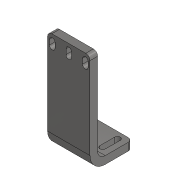
# Autodesk Inventor part: TL20240701-10200AT-005
Saved by Autodesk Inventor 2022.5 (Build 265521000, 521)
## iProperties
Category: ANTI BACK ASSY
Company: 현대트랜시스(대유)
RuleStatus: InUse
Part Number: TL20240701-10200AT-005
Project: SW-PJT
Checked By: 김형민
Engr Approved By: 김시현
User Status: 1
Material: SS400
Description: 0
Document SubType Name: Modeling
Mfg Approved By: 호상태
Designer: USER106
Stock Number: 005
Density: 7.85 g/cm^3
Appearance: Plating Zinc White
Detail Description: Processed products
Title: BRACKET
Subject: SW차종 시트조립라인
Author: USER106
Revision Number: A
Autodesk Inventor part; units mm, degrees
ref_plane "YZ Plane" through (0, 0, 0) normal (1, 0, 0) x (0, 1, 0)
ref_plane "XZ Plane" through (0, 0, 0) normal (0, 1, 0) x (-1, 0, 0)
ref_plane "XY Plane" through (0, 0, 0) normal (0, 0, 1) x (1, 0, 0)
sketch "Sketch2" plane through (0, 0, 0) normal (1, 0, 0) x (0, 1, 0)
  line L0 (-25, 60) -> (-25, -60)
  line L1 (-25, -60) -> (25, -60)
  line L2 (-16, 60) -> (-16, -51)
  line L3 (-16, -51) -> (25, -51)
  line L4 (-16, 60) -> (-25, 60)
  line L5 (25, -60) -> (25, -51)
  point P0 (0, 0)
  point P1 (-25, 0)
  point P2 (0, -60)
  dimension "d1" = 120
  dimension "d2" = 50
  dimension "t" = 9
  constraints: 12 end point, 2 midpoint, 2 perpendicular, 2 vertical, 1 horizontal, 1 horizontal alignment, 1 vertical alignment, 1 other
  measures "d1" distance of L0.start L0.end
  measures "d2" distance of L0.end L1.end
  measures "t" distance between parallel lines of L0 L2
extrude "Extrusion1" add sketch "Sketch2" along normal mid plane 50
fillet "Fillet1" radius 9 1 edges at (0, -16, -51)
fillet "Fillet1" radius 18 1 edges at (0, -25, -60)
sketch "Sketch3" plane through (-25, -25, 60) normal (0, -1, 0) x (1, 0, 0)
  line L0 (50, 0) -> (0, 0) projected
  line L1 (0, -102) -> (0, 0) projected
  line L2 (50, 0) -> (50, -102) projected
  line L3 (5.5, -13) -> (5.5, -7) construction
  line L4 (8.8, -13) -> (8.8, -7)
  line L5 (2.2, -7) -> (2.2, -13)
  arc A0 (2.2, -13) -> (8.8, -13) centre (5.5, -13) ccw
  arc A1 (8.8, -7) -> (2.2, -7) centre (5.5, -7) ccw
  line L6 (25, -13) -> (25, -7) construction
  line L7 (28.3, -13) -> (28.3, -7)
  line L8 (21.7, -7) -> (21.7, -13)
  arc A2 (21.7, -13) -> (28.3, -13) centre (25, -13) ccw
  arc A3 (28.3, -7) -> (21.7, -7) centre (25, -7) ccw
  line L9 (44.5, -13) -> (44.5, -7) construction
  line L10 (47.8, -13) -> (47.8, -7)
  line L11 (41.2, -7) -> (41.2, -13)
  arc A4 (41.2, -13) -> (47.8, -13) centre (44.5, -13) ccw
  arc A5 (47.8, -7) -> (41.2, -7) centre (44.5, -7) ccw
  point P0 (25, -60)
  point P1 (5.5, -10)
  point P2 (25, -10)
  point P3 (44.5, -10)
  dimension "d8" = 10
  dimension "d9" = 5.5
  dimension "d10" = 5.5
  dimension "d11" = 39
  dimension "d12" = 19.5
  dimension "d29" = 3
  dimension "d30" = 6.6
  dimension "d31" = 6.6
  constraints: 24 end point, 12 point on circle, 12 tangent, 6 centre point, 5 parallel, 3 midpoint, 3 vertical, 2 horizontal alignment, 1 equal radius
  measures "d8" distance from line of L0 point (5.5, -10)
  measures "d9" distance from line of point (5.5, -10) L1
  measures "d10" distance from line of point (44.5, -10) L2
  measures "d11" distance of point (44.5, -10) point (5.5, -10)
  measures "d12" distance of point (25, -10) point (5.5, -10)
  measures "d29" distance of point (5.5, -10) L3.end
  measures "d30" diameter of A1
  measures "d31" diameter of A3
sketch "Sketch4" plane through (-25, 25, -51) normal (0, 0, 1) x (1, 0, 0)
  line L0 (10, -7.5) -> (10, -25) construction
  line L1 (13.3, -7.5) -> (13.3, -25)
  line L2 (6.7, -25) -> (6.7, -7.5)
  arc A0 (13.3, -7.5) -> (6.7, -7.5) centre (10, -7.5) ccw
  arc A1 (6.7, -25) -> (13.3, -25) centre (10, -25) ccw
  line L3 (0, -32) -> (0, 0) projected
  line L4 (0, 0) -> (50, 0) projected
  line L5 (40, -7.5) -> (40, -25) construction
  line L6 (43.3, -7.5) -> (43.3, -25)
  line L7 (36.7, -25) -> (36.7, -7.5)
  arc A2 (43.3, -7.5) -> (36.7, -7.5) centre (40, -7.5) ccw
  arc A3 (36.7, -25) -> (43.3, -25) centre (40, -25) ccw
  point P0 (25, -25)
  point P1 (10, -16.25)
  point P2 (40, -16.25)
  dimension "d21" = 10
  dimension "d22" = 17.5
  dimension "d24" = 6.6
  dimension "d27" = 30
  dimension "d28" = 7.5
  constraints: 16 end point, 8 point on circle, 8 tangent, 4 centre point, 3 parallel, 2 midpoint, 2 vertical, 1 equal radius, 1 horizontal alignment
  measures "d21" distance between parallel lines of L0 L3
  measures "d22" distance of L0.start L0.end
  measures "d24" distance between parallel lines of L1 L2
  measures "d27" distance between parallel lines of L0 L5
  measures "d28" distance from line of L0.start L4
extrude "Extrusion2" cut sketch "Sketch4" along normal through all both and the other way through all
extrude "Extrusion3" cut sketch "Sketch3" along normal through all both and the other way through all
fillet "Fillet2" radius 5 4 edges at (-25, -20.5, 60) (25, -20.5, 60) (25, 25, -55.5) (-25, 25, -55.5)
equation "\"d6\" = t"
equation "\"d7\" = 2 * t"
equation "\"d10\" = d9"
equation "\"d12\" = 0.5 * d11"
body "Solid1"
